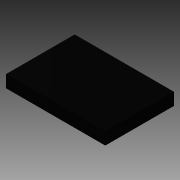
# Autodesk Inventor part: PCA9534PW
Saved by Autodesk Inventor 2015 SP1 (Build 190203100, 203)
## iProperties
Created: 2015-10-19
Part Number: PCA9534PW
Material: Generic
Document SubType Name: Modeling
Designer: Kartikye
Density: 1 g/cm^3
Appearance: SOP65P640X110-16N, PCA9534PW
Author: Kartikye
Autodesk Inventor part; units mm, degrees
ref_plane "YZ Plane" through (0, 0, 0) normal (1, 0, 0) x (0, 1, 0)
ref_plane "XZ Plane" through (0, 0, 0) normal (0, 1, 0) x (-1, 0, 0)
ref_plane "XY Plane" through (0, 0, 0) normal (0, 0, 1) x (1, 0, 0)
sketch "SOP65P640X110-16N, PCA9534PW_116" plane through (0, 0, 0) normal (0, 0, 1) x (1, 0, 0)
  line L0 (-3.9116, 2.794) -> (4.1656, 2.794)
  line L1 (4.1656, 2.794) -> (4.1656, -2.794)
  line L2 (4.1656, -2.794) -> (-3.9116, -2.794)
  line L3 (-3.9116, -2.794) -> (-3.9116, 2.794)
  constraints: 8 end point
extrude "Extrusion1" add sketch "SOP65P640X110-16N, PCA9534PW_116" along normal blind 1
body "Solid1"
